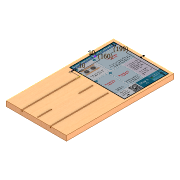
# Autodesk Inventor part: metrsync-platform-210
Saved by Autodesk Inventor 2020 (Build 240168000, 168)
## iProperties
Created: 2021-06-22
Part Number: metrsync-platform-210
Material: Generic
Document SubType Name: Modeling
Designer: Aidan Lee
Density: 1 g/cm^3
Appearance: Cherry - Natural Low Gloss
Author: Aidan Lee
Autodesk Inventor part; units mm, degrees
ref_plane "YZ Plane" through (0, 0, 0) normal (1, 0, 0) x (0, 1, 0)
ref_plane "XZ Plane" through (0, 0, 0) normal (0, 1, 0) x (-1, 0, 0)
ref_plane "XY Plane" through (0, 0, 0) normal (0, 0, 1) x (1, 0, 0)
sketch "Sketch2" plane through (0, 0, 0) normal (0, 0, 1) x (1, 0, 0)
  line L0 (0, 0) -> (219, 0)
  line L1 (219, 0) -> (219, 18)
  line L2 (219, 18) -> (0, 18)
  line L3 (0, 18) -> (0, 0)
  dimension "d0" = 18
  dimension "d1" = 219
  constraints: 8 end point, 2 parallel, 1 horizontal, 1 perpendicular
  measures "d0" distance of L2.end L0.start
  measures "d1" distance of L0.start L0.end
extrude "Extrusion1" add sketch "Sketch2" against normal blind 390
sketch "Sketch4" plane through (0, 18, 0) normal (0, 1, 0) x (1, 0, 0)
  line L0 (219, 0) -> (0, 0) projected
  line L1 (0, 0) -> (0, 390) projected
  line L2 (108, 5) -> (111, 5)
  line L3 (111, 5) -> (111, 205)
  line L4 (111, 205) -> (108, 205)
  line L5 (159.5, 0) -> (162.5, 0)
  line L6 (162.5, 0) -> (162.5, 210)
  line L7 (162.5, 210) -> (159.5, 210)
  line L8 (159.5, 210) -> (159.5, 0)
  line L9 (0, 0) -> (219, 0) construction
  line L10 (109.5, 0) -> (109.5, -15.4938) construction
  line L11 (219, 0) -> (219, 390) construction
  line L12 (59.5, 0) -> (56.5, 0)
  line L13 (56.5, 0) -> (56.5, 210)
  line L14 (56.5, 210) -> (59.5, 210)
  line L15 (59.5, 210) -> (59.5, 0)
  line L16 (108, 155) -> (111, 155)
  line L17 (111, 155) -> (111, 55)
  line L18 (111, 55) -> (108, 55)
  line L19 (108, 205) -> (108, 155)
  line L20 (108, 55) -> (108, 5)
  point P0 (109.5, 5)
  point P1 (111, 105)
  point P2 (159.5, 105)
  point P3 (56.5, 0)
  point P4 (59.5, 0)
  dimension "d4" = 3
  dimension "d6" = 210
  dimension "d8" = 3
  dimension "d19" = 200
  dimension "d20" = 100
  dimension "d21" = 50
  dimension "d22" = 50
  constraints: 34 end point, 6 midpoint, 6 parallel, 4 symmetric about line, 3 horizontal, 3 perpendicular, 2 point on line, 1 collinear, 1 horizontal alignment, 1 vertical, 1 vertical alignment
  measures "d4" distance of L6.end L7.end
  measures "d6" distance of L5.end L6.end
  measures "d8" distance of L3.end L4.end
  measures "d19" distance of L2.end L3.end
  measures "d20" distance between parallel lines of L8 L15
  measures "d21" distance from line of point (109.5, 5) L18
  measures "d22" distance of L3.end L16.end
extrude "Extrusion2" cut sketch "Sketch4" against normal blind 5
sketch "Sketch5" plane through (0, 18, -390) normal (0, 1, 0) x (1, 0, 0)
  line L0 (10, -170) -> (209, -170)
  line L1 (209, -170) -> (209, -10)
  line L2 (209, -10) -> (10, -10)
  line L3 (10, -10) -> (10, -170)
  line L4 (22.9605, -180) -> (22.9605, 0) construction
  line L5 (0, -390) -> (0, 0) construction
  line L6 (0, 0) -> (219, 0) construction
  line L7 (10, -170) -> (9.9883, -10.0145) construction
  line L8 (9.9883, -10.0145) -> (209, -10) construction
  line L9 (209, -10) -> (209.0117, -169.9855) construction
  line L10 (209.0117, -169.9855) -> (10, -170) construction
  point P0 (56.5, -180)
  point P1 (22.9605, -90)
  point P2 (10, -90)
  point P3 (109.5, -10)
  point P4 (109.5, 0)
  dimension "d15" = 10
  dimension "d16" = 10
  dimension "d17" = 160
  dimension "d18" = 199
  constraints: 10 end point, 4 midpoint, 3 horizontal alignment, 2 coincident, 2 parallel, 1 horizontal, 1 perpendicular, 1 vertical, 1 vertical alignment, 2 other
  measures "d15" distance from line of L0 point (56.5, -180)
  measures "d16" distance between parallel lines of L5 L3
  measures "d17" distance of L2.end L0.start
  measures "d18" distance of L1.end L2.end
body "Solid1"
